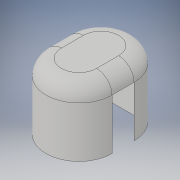
# Autodesk Inventor part: top
Saved by Autodesk Inventor 2019 (Build 230136000, 136)
## iProperties
Created: 2020-11-05
Part Number: top
Material: Generic
Document SubType Name: Modeling
Designer: Mike
Density: 1 g/cm^3
Appearance: Default
Author: Mike
Autodesk Inventor part; units mm, degrees
ref_plane "YZ Plane" through (0, 0, 0) normal (1, 0, 0) x (0, 1, 0)
ref_plane "XZ Plane" through (0, 0, 0) normal (0, 1, 0) x (-1, 0, 0)
ref_plane "XY Plane" through (0, 0, 0) normal (0, 0, 1) x (1, 0, 0)
sketch "Sketch1" plane through (0, 0, 0) normal (0, 1, 0) x (-1, 0, 0)
  line L0 (0, 0) -> (-30, 0)
  line L1 (-30, 0) -> (-30, -30)
  line L2 (-30, -30) -> (0, -30)
  line L3 (0, -30) -> (0, 0)
  dimension "d0" = 30
  dimension "d1" = 30
  constraints: 8 end point, 2 parallel, 1 horizontal, 1 perpendicular
  measures "d0" distance of L2.end L1.end
  measures "d1" distance of L1.end L0.end
extrude "Extrusion1" add sketch "Sketch1" along normal blind 7
fillet "Fillet1" radius 10 4 edges at (30, 3.5, -30) (0, 3.5, -30) (0, 3.5, 0) (30, 3.5, 0)
sketch "Sketch2" plane through (0, 7, 0) normal (0, 1, 0) x (1, 0, 0)
  line L0 (0, 35) -> (30, 35)
  line L1 (30, 35) -> (30, -5)
  line L2 (30, -5) -> (0, -5)
  line L3 (0, -5) -> (0, 35)
  line L4 (20, 30) -> (10, 30) projected
  line L5 (10, 0) -> (20, 0) projected
  line L6 (30, 10) -> (30, 20) projected
  line L7 (0, 20) -> (0, 10) projected
  arc A0 (20, 0) -> (30, 10) centre (20, 10) ccw projected
  line L8 (30, 10) -> (30, 20) projected
  arc A1 (30, 20) -> (20, 30) centre (20, 20) ccw projected
  line L9 (20, 30) -> (10, 30) projected
  arc A2 (10, 30) -> (0, 20) centre (10, 20) ccw projected
  line L10 (0, 20) -> (0, 10) projected
  arc A3 (0, 10) -> (10, 0) centre (10, 10) ccw projected
  line L11 (10, 0) -> (20, 0) projected
  point P0 (0, 0)
  dimension "d5" = 5
  dimension "d6" = 5
  dimension "d7" = 0
  dimension "d8" = 0
  constraints: 8 end point, 2 parallel, 1 horizontal, 1 perpendicular
  measures "d5" distance between parallel lines of L0 L4
  measures "d6" distance between parallel lines of L2 L5
  measures "d7" distance between parallel lines of L1 L6
  measures "d8" distance between parallel lines of L7 L3
extrude "Extrusion2" add sketch "Sketch2" against normal blind 30 contours L0 L1 A1 L4 A2 L3 | A3 L5 A0 L1 L2 L3
fillet "Fillet2" radius 15 4 edges at (30, -8, -35) (0, -8, 5) (0, -8, -35) (30, -8, 5)
fillet "Fillet3" radius 7 8 edges at (0, 7, -15) (4.3934, 7, -30.6066) (15, 7, -35) (25.6066, 7, -30.6066) (30, 7, -15) (4.3934, 7, 0.6066) (15, 7, 5) (25.6066, 7, 0.6066)
equation "\"d6\" = d5"
body "Solid1"
